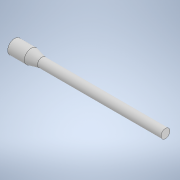
# Autodesk Inventor part: Scope
Saved by Autodesk Inventor 2021 (Build 250183000, 183)
## iProperties
Created: 2024-08-02
Part Number: Scope
Material: Generic
Document SubType Name: Modeling
Designer: Lukas
Density: 1 g/cm^3
Appearance: Default
Author: Lukas
Autodesk Inventor part; units mm, degrees
ref_plane "YZ Plane" through (0, 0, 0) normal (1, 0, 0) x (0, 1, 0)
ref_plane "XZ Plane" through (0, 0, 0) normal (0, 1, 0) x (-1, 0, 0)
ref_plane "XY Plane" through (0, 0, 0) normal (0, 0, 1) x (1, 0, 0)
sketch "Sketch2" plane through (0, 0, 0) normal (0, 0, 1) x (1, 0, 0)
  line L0 (-135, 12.5) -> (-135, 0)
  line L1 (-135, 0) -> (135, 0)
  line L2 (135, 0) -> (135, 8)
  line L3 (135, 8) -> (-86, 8)
  line L4 (-86, 8) -> (-105, 12.5)
  line L5 (-105, 12.5) -> (-135, 12.5)
  point P0 (0, 0)
  dimension "d3" = 270
  dimension "d4" = 12.5
  dimension "d5" = 8
  dimension "d6" = 30
  dimension "d7" = 19
  constraints: 12 end point, 2 midpoint, 2 perpendicular, 1 parallel, 1 vertical
  measures "d3" distance of L0.end L1.end
  measures "d4" distance of L0.start L0.end
  measures "d5" distance between parallel lines of L1 L3
  measures "d6" distance of L4.end L0.start
  measures "d7" horizontal distance of L3.end L4.end
revolve "Revolution1" add sketch "Sketch2" angle 360 about axis through (-135, 0, 0) along (1, 0, 0)
body "Solid2"
